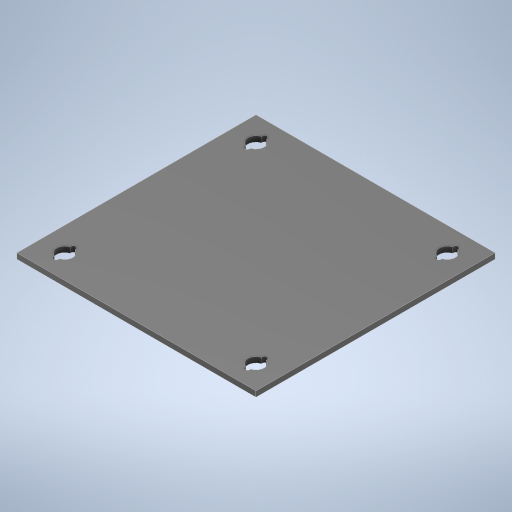
# Autodesk Inventor part: SUSTAINA-POWER-INPUT-BORAD
Saved by Autodesk Inventor 2024.2 (Build 282272000, 272)
## iProperties
Created: 2024-02-11
Part Number: SUSTAINA-POWER-INPUT-BORAD
Material: CFRP
Document SubType Name: Modeling
Designer: Masato Kubotera
Density: 1.43 g/cm^3
Appearance: Smooth - Black
Vendor: JLCPCB
Author: Masato Kubotera
Autodesk Inventor part; units mm, degrees
ref_plane "YZ Plane" through (0, 0, 0) normal (1, 0, 0) x (0, 1, 0)
ref_plane "XZ Plane" through (0, 0, 0) normal (0, 1, 0) x (-1, 0, 0)
ref_plane "XY Plane" through (0, 0, 0) normal (0, 0, 1) x (1, 0, 0)
sketch "Sketch1" plane through (0, 0, 0) normal (0, 0, 1) x (1, 0, 0)
  line L0 (35, 35) -> (-35, 35)
  line L1 (-35, 35) -> (-35, -35)
  line L2 (-35, -35) -> (35, -35)
  line L3 (35, -35) -> (35, 35)
  line L4 (35, 35) -> (-35, -35) construction
  line L5 (-35, 35) -> (35, -35) construction
  line L6 (-28, -28) -> (28, -28) construction
  line L7 (28, -28) -> (28, 28) construction
  line L8 (28, 28) -> (-28, 28) construction
  line L9 (-28, 28) -> (-28, -28) construction
  line L10 (-28, -28) -> (28, 28) construction
  line L11 (28, -28) -> (-28, 28) construction
  circle A0 centre (28, 28) radius 2.4
  arc A1 (30.2895, 27.2801) -> (30.2895, 28.7199) centre (30.5, 28) ccw
  line L12 (0, 35) -> (0, -35) construction
  line L13 (35, 0) -> (-35, 0) construction
  circle A2 centre (28, -28) radius 2.4
  arc A3 (30.2895, -28.7199) -> (30.2895, -27.2801) centre (30.5, -28) ccw
  line L14 (0, -35) -> (0, 35) construction
  circle A4 centre (-28, 28) radius 2.4
  arc A5 (-30.2895, 28.7199) -> (-30.2895, 27.2801) centre (-30.5, 28) ccw
  circle A6 centre (-28, -28) radius 2.4
  arc A7 (-30.2895, -27.2801) -> (-30.2895, -28.7199) centre (-30.5, -28) ccw
  arc A8 (25.7105, 28.7199) -> (25.7105, 27.2801) centre (25.5, 28) ccw
  arc A9 (25.7105, -27.2801) -> (25.7105, -28.7199) centre (25.5, -28) ccw
  arc A10 (-25.7105, 27.2801) -> (-25.7105, 28.7199) centre (-25.5, 28) ccw
  arc A11 (-25.7105, -28.7199) -> (-25.7105, -27.2801) centre (-25.5, -28) ccw
  point P0 (0, 0)
  point P1 (31.25, 28)
  point P2 (24.75, 28)
  dimension "d0" = 70
  dimension "d1" = 70
  dimension "d2" = 4.8
  dimension "d4" = 1.5
  dimension "d5" = 14
  dimension "d6" = 14
  dimension "d9" = 56
  dimension "d10" = 56
  dimension "d11" = 6.5
  constraints: 30 end point, 26 point on circle, 26 symmetric about line, 12 centre point, 8 midpoint, 4 parallel, 2 horizontal, 2 perpendicular, 1 coincident, 1 point on line, 10 other
  measures "d0" distance of L2.end L1.end
  measures "d1" distance of L1.end L0.end
  measures "d2" diameter of A0
  measures "d4" diameter of A1
  measures "d5" diameter of L3 L7
  measures "d6" diameter of L0 L8
  measures "d9" distance of L6.end L7.end
  measures "d10" distance of L7.end L8.end
  measures "d11" distance of point (31.25, 28) point (24.75, 28)
extrude "Extrusion1" add sketch "Sketch1" along normal blind 1.6
body "Solid1"
